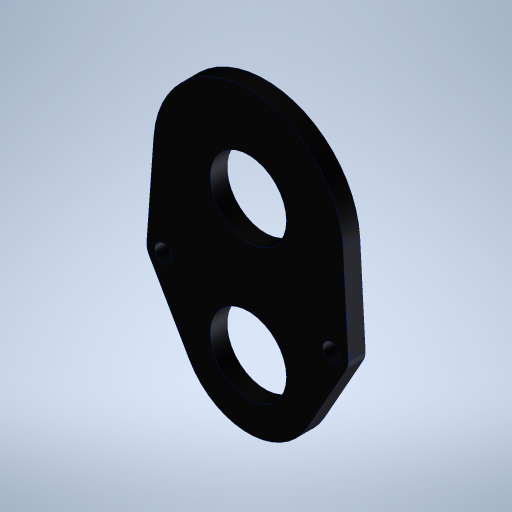
# Autodesk Inventor part: BottomPlate
Saved by Autodesk Inventor 2024 (Build 280153000, 153)
## iProperties
Created: 2024-07-07
Part Number: BottomPlate
Material: Aluminum 6061
Document SubType Name: Modeling
Designer: Danielle
Density: 2.7 g/cm^3
Appearance: Aluminum - Flat
Author: Danielle
Autodesk Inventor part; units mm, degrees
ref_plane "YZ Plane" through (0, 0, 0) normal (1, 0, 0) x (0, 1, 0)
ref_plane "XZ Plane" through (0, 0, 0) normal (0, 1, 0) x (-1, 0, 0)
ref_plane "XY Plane" through (0, 0, 0) normal (0, 0, 1) x (1, 0, 0)
sketch "Sketch1" plane through (0, 0, 0) normal (0, 0, 1) x (1, 0, 0)
  circle A0 centre (0, 0) radius 14.2875
  circle A1 centre (0, 0) radius 20.32 construction
  circle A2 centre (0, 50.8) radius 30.48 construction
  circle A3 centre (0, 50.8) radius 14.2875
  circle A4 centre (0, 50.8) radius 35.56 construction
  line L0 (0, 81.28) -> (0, 86.36)
  circle A5 centre (0, 0) radius 25.4 construction
  line L1 (0, 20.32) -> (0, 25.4) construction
  circle A6 centre (-31.7808, 17.1604) radius 6.35 construction
  circle A7 centre (31.1821, 16.6047) radius 6.35 construction
  line L2 (-27.42, 21.7763) -> (-24.4204, 24.9513) construction
  line L3 (-26.1933, 14.1434) -> (-22.3499, 12.0681) construction
  line L4 (26.8213, 11.9889) -> (23.8217, 8.8139) construction
  line L5 (26.9034, 21.2968) -> (23.9604, 24.5243) construction
  circle A8 centre (-31.7808, 17.1604) radius 3.2639
  circle A9 centre (31.1821, 16.6047) radius 3.2639
  line L6 (-37.2911, 14.0047) -> (-22.0413, -12.6231)
  line L7 (36.718, 13.494) -> (22.1435, -12.4429)
  line L8 (-38.1134, 17.6293) -> (-35.4629, 53.4258)
  line L9 (37.522, 16.9618) -> (35.5037, 52.7995)
  arc A10 (-38.1134, 17.6293) -> (-37.2911, 14.0047) centre (-31.7808, 17.1604) ccw
  arc A11 (36.718, 13.494) -> (37.522, 16.9618) centre (31.1821, 16.6047) ccw
  arc A12 (35.5037, 52.7995) -> (-35.4629, 53.4258) centre (0, 50.8) ccw
  arc A13 (-22.0413, -12.6231) -> (22.1435, -12.4429) centre (0, 0) ccw
  dimension "d1" = 40.64
  dimension "d0" = 28.575
  dimension "d2" = 60.96
  dimension "d3" = 28.575
  dimension "d4" = 5.08
  dimension "d5" = 71.12
  dimension "d6" = 5.08
  dimension "d9" = 12.7
  dimension "d10" = 3.175
  dimension "d11" = 6.5278
  dimension "d12" = 6.5278
  constraints: 28 point on circle, 20 end point, 13 centre point, 12 tangent, 7 coincident, 7 point on line, 3 equal length, 3 equal radius, 2 vertical, 2 vertical alignment, 1 parallel, 3 other
  measures "d0" diameter of A0
  measures "d2" diameter of A2
  measures "d3" diameter of A3
  measures "d4" distance of L0.end L0.start
  measures "d5" diameter of A4
  measures "d6" distance of L1.start L1.end
  measures "d9" diameter of A6
  measures "d10" vertical distance of L2.start L2.end
  measures "d11" diameter of A8
  measures "d12" diameter of A9
extrude "Extrusion2" add sketch "Sketch1" along normal blind 6.35
body "Solid2"
